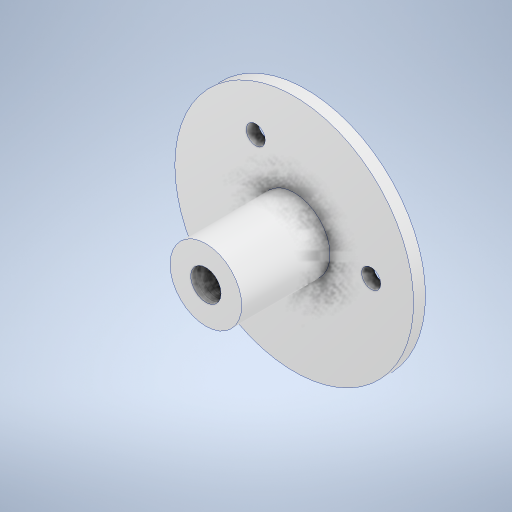
# Autodesk Inventor part: Test flange
Saved by Autodesk Inventor 2023 (Build 270158000, 158)
## iProperties
Created: 2022-06-23
Part Number: Test flange
Material: Aluminum 6061
Document SubType Name: Sheet Metal
Designer: earls
Density: 2.7 g/cm^3
Appearance: Aluminum - Flat
Sheet Metal Rule: Default_mm
Author: earls
Autodesk Inventor part; units mm, degrees
ref_plane "YZ Plane" through (0, 0, 0) normal (1, 0, 0) x (0, 1, 0)
ref_plane "XZ Plane" through (0, 0, 0) normal (0, 1, 0) x (-1, 0, 0)
ref_plane "XY Plane" through (0, 0, 0) normal (0, 0, 1) x (1, 0, 0)
sketch "Sketch1" plane through (0, 0, 0) normal (0, 0, 1) x (1, 0, 0)
  circle A0 centre (0, 0) radius 100
  line L0 (0, 100) -> (86.6025, 50)
  line L1 (86.6025, 50) -> (86.6025, -50)
  line L2 (86.6025, -50) -> (0, -100)
  line L3 (0, -100) -> (-86.6025, -50)
  line L4 (-86.6025, -50) -> (-86.6025, 50)
  line L5 (-86.6025, 50) -> (0, 100)
  circle A1 centre (0, 0) radius 50
  circle A2 centre (0, 0) radius 15
  circle A3 centre (0, 0) radius 6.35
  circle A4 centre (32.256, 0) radius 4
  circle A5 centre (-16.128, 27.9345) radius 4
  circle A6 centre (-16.128, -27.9345) radius 4
  dimension "d0" = 200
  dimension "d1" = 100
  dimension "d2" = 30
  dimension "d3" = 12.7
  dimension "d4" = 8
  dimension "d7" = 360
  constraints: 12 end point, 6 centre point, 5 coincident, 1 horizontal alignment, 1 vertical alignment, 22 other
  measures "d1" diameter of A1
  measures "d2" diameter of A2
  measures "d3" diameter of A3
  measures "d4" diameter of A4
extrude "Plate1" add sketch "Sketch1" against normal blind 5 contours A1 | A2 | A3
extrude "Extrusion1" add sketch "Sketch1" along normal blind 37 contours A2
thread "Thread1" size "M14x2" class "6H" standard "ANSI Metric M Profile" full length
equation "\"d9\" = Thickness"
equation "\"BendRadius\" = Thickness"
equation "\"BendReliefWidth\" = Thickness"
equation "\"BendReliefDepth\" = 0.5 * Thickness"
equation "\"TransitionRadius\" = BendRadius"
equation "\"JacobiRadiusSize\" = BendRadius"
equation "\"GapSize\" = Thickness"
equation "\"Thickness\" = 5"
body "Solid1"
